Autodesk Fusion 360 part; units mm, degrees
(part 2 of 2)
equation "d28 = bd / 2"
equation "d32 = bd / 2"
equation "d34 = bd * 3"
equation "d36 = bd"
equation "d38 = t"
equation "d48 = -t"
equation "d50 = -t"
equation "d63 = t"
equation "d68 = -t"
equation "d70 = -t"
equation "d80 = t"
equation "d87 = -t"
equation "d125 = -t"
equation "d127 = -t"
equation "d129 = -t"
equation "d133 = -t"
equation "d135 = -t"
named bodies: "Base", "Front", "Back", "Right Side (Master)", "Side", "Left Side", "Middle Side", "Left Ramp (Master)", "Right Ramp", "Left Ramp (Master) (1)", "Right Ramp (1)", "Right Side", "Right Side (1)"
